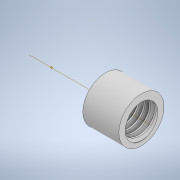
# Autodesk Inventor part: 1aThreadsV04-1_2x13-internalTest
Saved by Autodesk Inventor 2021.1 (Build 251245010, 245A)
## iProperties
Created: 2020-10-17
Part Number: 1aThreadsV04-1_2x13-internalTest
Material: Generic
Document SubType Name: Modeling
Designer: robst
Density: 1 g/cm^3
Appearance: Default
Author: robst
Autodesk Inventor part; units mm, degrees
ref_plane "XZ Plane" through (0, 0, 0) normal (0, 1, 0) x (-1, 0, 0)
ref_plane "XY Plane" through (0, 0, 0) normal (0, 0, 1) x (1, 0, 0)
sketch "InternalThreadSketch" plane through (0, 0, 0) normal (0, 0, 1) x (1, 0, 0)
  line L0 (32.0205, 5.4) -> (32.6144, 6.4287)
  line L1 (32.7992, 6.4287) -> (33.3931, 5.4)
  arc A0 (32.7992, 6.4287) -> (32.6144, 6.4287) centre (32.7068, 6.3754) ccw
  line L2 (32.0205, 5.4) -> (31.4795, 5.4)
  line L3 (33.3931, 5.4) -> (33.9341, 5.4)
  line L4 (-6.7868, 0) -> (40.721, 0) projected
  line L5 (31.75, 5.4) -> (33.7038, 5.4) construction
  line L6 (33.7038, 5.4) -> (33.7038, 6.4821) construction
  line L7 (33.7038, 6.4821) -> (31.75, 6.4821) construction
  line L8 (31.75, 6.4821) -> (31.75, 5.4) construction
  line L9 (32.0205, 5.4) -> (33.3931, 5.4)
  point P0 (0, 0)
  dimension "d71" = 60
  dimension "d72" = 0.1067
  dimension "d73" = 0.541
  dimension "d75" = 6.4821
  dimension "d76" = 5.4
  dimension "d77" = 120
  dimension "d78" = 31.75
  dimension "d79" = 1.9539
  constraints: 18 end point, 3 collinear, 3 horizontal, 3 tangent, 2 parallel, 2 point on circle, 1 centre point, 1 midpoint, 1 perpendicular
  measures "d71" angle of L1 L0
  measures "d72" radius of A0
  measures "d73" distance of L0.start L2.end
  measures "d76" distance between parallel lines of L3 L4
  measures "d77" angle of L0 L2
  measures "d78" distance from line of L8 point (0, 0)
  measures "d79" distance between parallel lines of L6 L8
ref_plane "Work Plane1" through (31.75, 0, 0) normal (1, 0, 0) x (0, 1, 0)
sketch "Sketch4" plane through (31.75, 0, 0) normal (1, 0, 0) x (0, 1, 0)
  circle A0 centre (0, 0) radius 5.4
  circle A1 centre (0, 0) radius 7.94
  dimension "d93" = 10.8001
  dimension "d94" = 2.54
  constraints: 2 centre point, 2 coincident
  measures "d93" diameter of A0
  measures "d94" radial gap between concentric circles of A1 A0
extrude "Extrusion2" add sketch "Sketch4" against normal blind 12.7
coil "Coil3" sketch "InternalThreadSketch" operation cut axis through (-10, 0, 0) along (-1, 0, 0) pitch 1.9538 turns 8.5 hand right
equation "\"d71\" = threadAngle"
equation "\"d72\" = b1RootRadius"
equation "\"d73\" = b1CrestFlat"
equation "\"d75\" = b1MajorRadius"
equation "\"d76\" = b1MinorRadius"
equation "\"d79\" = pitch"
equation "\"d93\" = b1MinorDiameter"
equation "\"d105\" = pitch"
equation "\"threadAngle\" = 60deg"
equation "\"b1MajorDiameter\" = 12.96416"
equation "\"b1MajorRadius\" = 0.5 * b1MajorDiameter"
equation "\"b1MinorDiameter\" = 10.80008"
equation "\"b1RootRadius\" = 0.10668"
equation "\"b1MinorRadius\" = 0.5 * b1MinorDiameter"
equation "\"b1ThreadDepth\" = 1.08204"
equation "\"b1CrestFlat\" = 0.54102"
equation "\"pitch\" = 1.953846"
body "Solid2"
